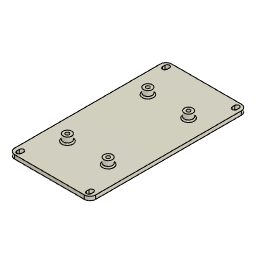
Lower Bay Tray - LM2596 with LED (Autodesk Fusion 360 design; units mm, degrees)
Autodesk Fusion 360 part; units mm, degrees
sketch "Sketch40" plane through (0, 0, 8) normal (0, 0, 1) x (1, 0, 0)
  circle A0 centre (65, 135) radius 1.4 construction
  circle A1 centre (65, 135) radius 3.4 construction
  circle A2 centre (10, 135) radius 1.4 construction
  circle A3 centre (10, 135) radius 3.4 construction
  circle A4 centre (-10, 135) radius 1.4 construction
  circle A5 centre (-10, 135) radius 3.4 construction
  circle A6 centre (-65, 135) radius 1.4 construction
  circle A7 centre (-65, 135) radius 3.4 construction
  circle A8 centre (-65, 20) radius 1.4 construction
  circle A9 centre (-65, 20) radius 3.4 construction
  circle A10 centre (-10, 20) radius 1.4 construction
  circle A11 centre (-10, 20) radius 3.4 construction
  circle A12 centre (10, 20) radius 1.4 construction
  circle A13 centre (10, 20) radius 3.4 construction
  circle A14 centre (65, 20) radius 1.4 construction
  circle A15 centre (65, 20) radius 3.4 construction
  line L0 (10, 135) -> (65, 135) construction
  line L1 (65, 135) -> (65, 20) construction
  line L2 (65, 20) -> (10, 20) construction
  line L3 (10, 20) -> (10, 135) construction
  line L4 (-10, 135) -> (-65, 135) construction
  line L5 (-65, 135) -> (-65, 20) construction
  line L6 (-65, 20) -> (-10, 20) construction
  line L7 (-10, 20) -> (-10, 135) construction
  arc A16 (-69.5, 20) -> (-65, 15.5) centre (-65, 20) ccw
  arc A17 (-10, 15.5) -> (-5.5, 20) centre (-10, 20) ccw
  arc A18 (-5.5, 135) -> (-10, 139.5) centre (-10, 135) ccw
  arc A19 (-65, 139.5) -> (-69.5, 135) centre (-65, 135) ccw
  line L8 (-69.5, 135) -> (-5.5, 135) construction
  line L9 (-5.5, 135) -> (-5.5, 20)
  line L10 (-10, 139.5) -> (-65, 139.5)
  line L11 (-10, 15.5) -> (-65, 15.5)
  line L12 (-69.5, 20) -> (-69.5, 135)
  line L13 (0, 0) -> (0, 50) construction
  line L14 (-66.8, 136) -> (-66.8, 134)
  arc A20 (-66.8, 134) -> (-63.2, 134) centre (-65, 134) ccw
  line L15 (-63.2, 134) -> (-63.2, 136)
  arc A21 (-63.2, 136) -> (-66.8, 136) centre (-65, 136) ccw
  line L16 (-65, 136) -> (-65, 134) construction
  arc A22 (-8.2, 136) -> (-11.8, 136) centre (-10, 136) ccw
  line L17 (-11.8, 136) -> (-11.8, 134)
  arc A23 (-11.8, 134) -> (-8.2, 134) centre (-10, 134) ccw
  line L18 (-8.2, 134) -> (-8.2, 136)
  line L19 (-5.5, 77.5) -> (-69.5, 77.5) construction
  arc A24 (-11.8, 19) -> (-8.2, 19) centre (-10, 19) ccw
  line L20 (-11.8, 19) -> (-11.8, 21)
  arc A25 (-8.2, 21) -> (-11.8, 21) centre (-10, 21) ccw
  line L21 (-8.2, 21) -> (-8.2, 19)
  arc A26 (-66.8, 19) -> (-63.2, 19) centre (-65, 19) ccw
  line L22 (-66.8, 19) -> (-66.8, 21)
  line L23 (-63.2, 21) -> (-63.2, 19)
  arc A27 (-63.2, 21) -> (-66.8, 21) centre (-65, 21) ccw
  line L24 (-37.5, 139.5) -> (-37.5, 15.5) construction
  point P0 (-65, 135)
  point P1 (-37.5, 77.5)
  dimension "d905" = 1.8
  dimension "d906" = 1.8
  dimension "d908" = 3.5
  dimension "d910" = 2
  constraint horizontal L0
  constraint vertical L1
  constraint horizontal L2
  constraint vertical L3
  constraint coincident A14.centre A15.centre
  constraint coincident A2.centre A3.centre
  constraint horizontal L4
  constraint vertical L5
  constraint horizontal L6
  constraint vertical L7
  constraint coincident A8.centre A9.centre
  constraint coincident A4.centre A5.centre
  constraint concentric A9 A16
  constraint concentric A11 A17
  constraint concentric A5 A18
  constraint concentric A7 A19
  constraint parallel L4 L8
  constraint tangent A17 L9
  constraint perpendicular L8 L9
  constraint tangent A19 L10
  constraint parallel L8 L10
  constraint tangent A16 L11
  constraint parallel L10 L11
  constraint tangent A19 L12
  constraint coincident L13.start origin
  constraint perpendicular L2 L13
  constraint tangent L14 A20
  constraint tangent A20 L15
  constraint parallel L14 L15
  constraint tangent L15 A21
  constraint tangent L14 A21
  constraint coincident L5 A20.centre
  constraint parallel L5 L16
  constraint coincident P0 A6.centre
  constraint midpoint L16 P0
  constraint tangent L17 A23
  constraint tangent A23 L18
  constraint parallel L17 L18
  constraint tangent A22 L18
  constraint tangent A22 L17
  constraint midpoint L9 L19.start
  constraint midpoint L12 L19.end
  constraint symmetric L14.start L19 A26.start
  constraint symmetric L14.end L19 L22.end
  constraint symmetric A20.end L19 L23.start
  constraint symmetric L15.end L19 A26.end
  constraint symmetric A20 L19 A27
  constraint symmetric A21 L19 A26
  constraint symmetric A22.end L19 A24.start
  constraint symmetric L17.end L19 L20.end
  constraint symmetric A22.start L19 A24.end
  constraint symmetric A23.end L19 A25.start
  constraint symmetric A22 L19 A24
  constraint symmetric A23 L19 A25
  constraint midpoint L10 L24.start
  constraint midpoint L11 L24.end
  constraint midpoint L24 P1
  measures "d905" radius of A21
  measures "d906" radius of A22
  measures "d908" distance of L10 A21.centre
  measures "d910" distance of A21.centre A20.centre
extrude "Extrude1" add sketch "Sketch40" along normal blind 3
sketch "Sketch1" plane through (0, 0, 11) normal (0, 0, 1) x (-1, 0, 0)
  arc A0 (63.2, -136) -> (66.8, -136) centre (65, -136) ccw
  line L0 (63.2, -136) -> (63.2, -134)
  arc A1 (66.8, -134) -> (63.2, -134) centre (65, -134) ccw
  line L1 (66.8, -134) -> (66.8, -136)
  arc A2 (66.8, -19) -> (63.2, -19) centre (65, -19) ccw
  line L2 (66.8, -19) -> (66.8, -21)
  arc A3 (63.2, -21) -> (66.8, -21) centre (65, -21) ccw
  line L3 (63.2, -21) -> (63.2, -19)
  line L4 (8.2, -136) -> (8.2, -134)
  arc A4 (11.8, -134) -> (8.2, -134) centre (10, -134) ccw
  line L5 (11.8, -134) -> (11.8, -136)
  arc A5 (8.2, -136) -> (11.8, -136) centre (10, -136) ccw
  arc A6 (11.8, -19) -> (8.2, -19) centre (10, -19) ccw
  line L6 (11.8, -19) -> (11.8, -21)
  arc A7 (8.2, -21) -> (11.8, -21) centre (10, -21) ccw
  line L7 (8.2, -21) -> (8.2, -19)
  arc A8 (10, -15.5) -> (5.5, -20) centre (10, -20) ccw
  line L8 (5.5, -20) -> (5.5, -135)
  arc A9 (5.5, -135) -> (10, -139.5) centre (10, -135) ccw
  line L9 (10, -139.5) -> (65, -139.5)
  arc A10 (65, -139.5) -> (69.5, -135) centre (65, -135) ccw
  line L10 (69.5, -135) -> (69.5, -20)
  arc A11 (69.5, -20) -> (65, -15.5) centre (65, -20) ccw
  line L11 (65, -15.5) -> (10, -15.5)
  line L12 (5.5, -77.5) -> (69.5, -77.5) construction
  line L13 (37.5, -77.5) -> (37.5, -15.5) construction
  line L14 (21.435, -45.75) -> (53.565, -45.75) construction
  line L15 (53.565, -45.75) -> (53.565, -109.25) construction
  line L16 (53.565, -109.25) -> (21.435, -109.25) construction
  line L17 (21.435, -109.25) -> (21.435, -45.75) construction
  line L18 (21.435, -45.75) -> (53.565, -109.25) construction
  line L19 (53.565, -45.75) -> (21.435, -109.25) construction
  circle A12 centre (21.435, -109.25) radius 1.4
  circle A13 centre (53.565, -109.25) radius 1.4
  circle A14 centre (21.435, -45.75) radius 1.4
  circle A15 centre (53.565, -45.75) radius 1.4
  circle A16 centre (53.565, -45.75) radius 3.4
  circle A17 centre (21.435, -45.75) radius 3.4
  circle A18 centre (21.435, -109.25) radius 3.4
  circle A19 centre (53.565, -109.25) radius 3.4
  point P0 (37.5, -77.5)
  dimension "d1" = 32.13
  dimension "d2" = 63.5
  dimension "d3" = 2.8
  dimension "d4" = 2.8
  dimension "d5" = 2.8
  dimension "d6" = 2.8
  dimension "d7" = 2
  dimension "d8" = 2
  dimension "d9" = 2
  dimension "d10" = 2
  constraint midpoint L8 L12.start
  constraint midpoint L10 L12.end
  constraint midpoint L12 P0
  constraint midpoint L11 L13.end
  constraint horizontal L14
  constraint perpendicular L14 L15
  constraint parallel L14 L16
  constraint parallel L15 L17
  constraint coincident L18 P0
  constraint coincident L19 P0
  constraint coincident P0 L13.start
  constraint coincident L16.end L17.start
  constraint coincident L15.end L16.start
  constraint coincident L14.start L17.end
  constraint coincident L14.end L15.start
  measures "d1" distance of L15.end L16.end
  measures "d2" distance of L14.end L15.end
  measures "d3" diameter of A12
  measures "d4" diameter of A13
  measures "d5" diameter of A14
  measures "d6" diameter of A15
extrude "Extrude2" add sketch "Sketch1" along normal blind 5 contours A16 | A17 | A18 | A19
fillet "Fillet1" radius 1 4 edges at (-18.2651, 44.5205, 11) (-50.3951, 44.5205, 11) (-18.2651, 108.0205, 11) (-50.3951, 108.0205, 11)
equation "d905 = large_m3 / 2"
equation "d906 = large_m3 / 2"
equation "large_m3 = 3.6 mm"
